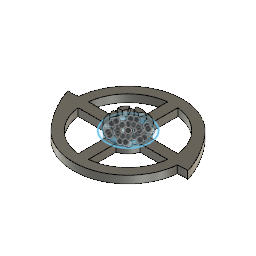
circular double tooth v9 (Autodesk Fusion 360 design; units mm, degrees)
Autodesk Fusion 360 part; units mm, degrees
note: some values were not read from the file. Set by a fixed rule: which sketch regions a step uses.
sketch "Sketch1" plane through (0, 0, 0) normal (0, 0, 1) x (1, 0, 0)
  circle A0 centre (0, 0) radius 2.95
  circle A1 centre (0, 0) radius 13.9
  circle A2 centre (0, 0) radius 50.5
  circle A3 centre (0, 0) radius 42.5
  line L0 (0, 0) -> (0, 50.5) construction
  line L1 (0, 0) -> (50, 0) construction
  line L2 (0, 0) -> (0, -50.5) construction
  line L3 (0, 0) -> (-50.5, 0) construction
  line L4 (0, -4) -> (-50.3413, -4)
  line L5 (0, 4) -> (-50.3413, 4)
  line L6 (0, 4) -> (50.3413, 4)
  line L7 (0, -4) -> (50.3413, -4)
  line L8 (-4, 0) -> (-4, 50)
  line L9 (4, 0) -> (4, 50)
  line L10 (4, 0) -> (4, -50)
  line L11 (-4, 0) -> (-4, -50)
  circle A4 centre (0, 0) radius 35
  spline S0 degree 5 poles (-50.3413, 4) (-50.1483, 3.3288) (-49.755, 2.0187) (-49.1428, 0.1498) (-48.2761, -2.1757) (-47.0702, -4.9467) (-45.6928, -7.7451) (-44.094, -10.7131) (-42.2399, -13.9102) (-40.1125, -17.3141) (-37.6988, -20.8633) (-35.5301, -23.7571) (-33.7651, -25.9282) (-32.5263, -27.3718) (-31.8913, -28.0927) knots 0 0 0 0 0 0 0.1 0.2 0.3 0.4 0.5 0.6 0.7 0.8 0.9 1 1 1 1 1 1
  line L12 (-51.0873, 6.594) -> (-49.5954, 1.406)
  line L13 (-33.7745, -25.9547) -> (-30.008, -30.2306)
  spline S1 degree 5 poles (-50.3413, 4) (-50.2904, 3.9577) (-50.1779, 3.8772) (-49.9773, 3.7688) (-49.645, 3.6492) (-49.1156, 3.5438) (-48.4657, 3.4848) (-47.6934, 3.4729) (-46.8065, 3.5051) (-45.8162, 3.5771) (-44.7343, 3.6845) (-43.8031, 3.7959) (-43.0704, 3.8929) (-42.5669, 3.9633) (-42.3113, 4) knots 0 0 0 0 0 0 0.1 0.2 0.3 0.4 0.5 0.6 0.7 0.8 0.9 1 1 1 1 1 1
  line L14 (-50.752, 4.3411) -> (-49.9307, 3.6589)
  line L15 (-43.3417, 3.852) -> (-41.281, 4.148)
  spline S2 degree 5 poles (50.3413, -4) (50.1483, -3.3288) (49.755, -2.0187) (49.1428, -0.1498) (48.2761, 2.1757) (47.0702, 4.9467) (45.6928, 7.7451) (44.094, 10.7131) (42.2399, 13.9102) (40.1125, 17.3141) (37.6988, 20.8633) (35.5301, 23.7571) (33.7651, 25.9282) (32.5263, 27.3718) (31.8913, 28.0927) knots 0 0 0 0 0 0 0.1 0.2 0.3 0.4 0.5 0.6 0.7 0.8 0.9 1 1 1 1 1 1
  line L16 (51.0873, -6.594) -> (49.5954, -1.406)
  line L17 (33.7745, 25.9547) -> (30.008, 30.2306)
  spline S3 degree 5 poles (50.3413, -4) (50.2904, -3.9577) (50.1779, -3.8772) (49.9773, -3.7688) (49.645, -3.6492) (49.1156, -3.5438) (48.4657, -3.4848) (47.6934, -3.4729) (46.8065, -3.5051) (45.8162, -3.5771) (44.7343, -3.6845) (43.8031, -3.7959) (43.0704, -3.8929) (42.5669, -3.9633) (42.3113, -4) knots 0 0 0 0 0 0 0.1 0.2 0.3 0.4 0.5 0.6 0.7 0.8 0.9 1 1 1 1 1 1
  line L18 (50.752, -4.3411) -> (49.9307, -3.6589)
  line L19 (43.3417, -3.852) -> (41.281, -4.148)
  point P0 (-45, -9)
  point P1 (-48.5, 3.5)
  point P2 (45, 9)
  point P3 (48.5, -3.5)
  dimension "d1" = 5.9
  dimension "d2" = 27.8
  dimension "d3" = 101
  dimension "d4" = 85
  dimension "d5" = 4
  dimension "d6" = 4
  dimension "d7" = 70
  constraint coincident A0.centre A1.centre
  constraint coincident A2 L0.end
  constraint vertical L0
  constraint perpendicular L0 L1
  constraint coincident A2 L2.end
  constraint vertical L2
  constraint coincident A2 L3.end
  constraint perpendicular L2 L3
  constraint coincident L2 L4.start
  constraint coincident A2 L4.end
  constraint perpendicular L2 L4
  constraint symmetric L3 L4.start L5.start
  constraint symmetric L3 L4.end L5.end
  constraint symmetric L0 L4.start L7.start
  constraint symmetric L0 L4.end L7.end
  constraint symmetric L0 L5.start L6.start
  constraint symmetric L0 L5.end L6.end
  constraint coincident L3 L8.start
  constraint perpendicular L3 L8
  constraint symmetric L0 L8.start L9.start
  constraint symmetric L0 L8.end L9.end
  constraint symmetric L1 L8.start L11.start
  constraint symmetric L1 L8.end L11.end
  constraint symmetric L1 L9.start L10.start
  constraint symmetric L1 L9.end L10.end
  constraint concentric A2 A4
  constraint midpoint L5.end L12
  constraint midpoint S0.end L13
  constraint coincident L5 S1.end
  constraint coincident A3 S1.end
  constraint midpoint L5.end L14
  constraint midpoint S1.end L15
  constraint coincident A3 S0.end
  constraint tangent A3 L13
  measures "d1" diameter of A0
  measures "d2" diameter of A1
  measures "d3" diameter of A2
  measures "d4" diameter of A3
  measures "d5" distance of L3 L4
  measures "d6" distance of L0 L8
  measures "d7" diameter of A4
extrude "Extrude1" add sketch "Sketch1" along normal mid plane 6 contours A1 L6 L7 L9 L10 | A1 L6 L7 A4 | A1 L6 L9 | A1 L7 L10 | A1 L5 L6 L8 L9 | A1 L8 L9 A4 | L4 L5 L6 L7 L8 L9 L10 L11 | A3 L6 L9 A4 | A3 L6 L7 A4 | A1 L10 L11 A4 | A1 L4 L7 L10 L11 | A3 L7 L10 A4 | A1 L5 L8 | A3 L8 L9 A4 | A3 L6 S2 S3 | A3 L6 S2 | A1 L4 L11 | A3 L10 L11 A4 | A1 L4 L5 L8 L11 | A1 L4 L5 A4 | A3 L5 L8 A4 | A3 L4 L11 A4 | A3 L4 L5 A4 | A3 L4 S0 S1 | A3 L4 S0
ref_plane "WorkPlane1" through (0, 0, 3) normal (0, 0, 1) x (1, 0, 0)
sketch "Sketch2" plane through (0, 0.1618, 3) normal (0, 0, 1) x (1, 0, 0)
  line L0 (-2.034, -6.023) -> (-4.3462, -10.0278)
  spline S0 degree 3 poles (-10.8574, -1.65) (-10.8584, -1.65) (-10.8595, -1.6501) (-10.8605, -1.6503) (-10.862, -1.6506) (-10.8635, -1.6511) (-10.8648, -1.6519) (-10.8666, -1.6528) (-10.8681, -1.654) (-10.8696, -1.6558) (-10.8707, -1.6572) (-10.8716, -1.6587) (-10.8722, -1.6607) (-10.8729, -1.6626) (-10.8731, -1.6646) (-10.873, -1.6667) knots -0.08749 -0.08749 -0.08749 -0.08749 -0.077534 -0.077534 -0.077534 -0.062667 -0.062667 -0.062667 -0.04351 -0.04351 -0.04351 -0.027229 -0.027229 -0.027229 -0.010666 -0.010666 -0.010666 -0.010666
  spline S1 degree 3 poles (-1.5005, -6.1547) (-1.5145, -6.1513) (-1.5288, -6.1496) (-1.5432, -6.1497) (-1.5589, -6.1497) (-1.5744, -6.1518) (-1.5895, -6.1559) (-1.6081, -6.161) (-1.6256, -6.169) (-1.6416, -6.1796) (-1.6557, -6.189) (-1.6683, -6.2003) (-1.6791, -6.2132) (-1.6837, -6.2186) (-1.6878, -6.2242) (-1.6917, -6.2301) knots -0.077702 -0.077702 -0.077702 -0.077702 -0.063693 -0.063693 -0.063693 -0.048454 -0.048454 -0.048454 -0.029774 -0.029774 -0.029774 -0.013339 -0.013339 -0.013339 -0.006509 -0.006509 -0.006509 -0.006509
  arc A0 (-4.2907, -4.1005) -> (-1.4057, -5.7661) centre (0, 0) ccw
  arc A1 (-11.2693, -1.7216) -> (-7.1256, -8.8987) centre (0, 0) ccw
  circle A2 centre (0, 0) radius 16.7005
  spline S2 degree 3 poles (-4.3462, -10.0278) (-4.349, -10.0327) (-4.3517, -10.0376) (-4.357, -10.0477) (-4.3595, -10.0528) (-4.3635, -10.0611) (-4.3649, -10.0643) (-4.3677, -10.0705) (-4.3689, -10.0734) (-4.3717, -10.0801) (-4.3732, -10.0838) (-4.3775, -10.0951) (-4.3801, -10.1027) (-4.3954, -10.1509) (-4.402, -10.1935) (-4.4018, -10.2542) (-4.4007, -10.2718) (-4.3915, -10.3419) (-4.3744, -10.3946) (-4.3231, -10.4833) (-4.2929, -10.5203) (-4.2227, -10.5801) (-4.185, -10.6033) (-4.1437, -10.6203) knots -0.079764 -0.079764 -0.079764 -0.079764 -0.077736 -0.077736 -0.075667 -0.075667 -0.074396 -0.074396 -0.073245 -0.073245 -0.071774 -0.071774 -0.068877 -0.068877 -0.053423 -0.053423 -0.047168 -0.047168 -0.028481 -0.028481 -0.013393 -0.013393 0 0 0 0
  spline S3 degree 3 poles (-10.8574, -1.25) (-10.8623, -1.25) (-10.8672, -1.2501) (-10.8783, -1.2505) (-10.8845, -1.2508) (-10.8945, -1.2516) (-10.8984, -1.252) (-10.9058, -1.2528) (-10.9094, -1.2532) (-10.9175, -1.2543) (-10.9221, -1.255) (-10.9363, -1.2574) (-10.9458, -1.2594) (-11.0105, -1.2751) (-11.063, -1.2998) (-11.1532, -1.3685) (-11.1916, -1.4115) (-11.2435, -1.5046) (-11.2601, -1.5511) (-11.2742, -1.6405) (-11.2748, -1.6811) (-11.2693, -1.7216) knots -0.086203 -0.086203 -0.086203 -0.086203 -0.084433 -0.084433 -0.082213 -0.082213 -0.08081 -0.08081 -0.079512 -0.079512 -0.077841 -0.077841 -0.0743 -0.0743 -0.053753 -0.053753 -0.034336 -0.034336 -0.018768 -0.018768 -0.006485 -0.006485 -0.006485 -0.006485
  spline S4 degree 3 poles (-5.6965, -1.6656) (-5.7165, -1.5973) (-5.7489, -1.5333) (-5.8314, -1.4253) (-5.8791, -1.3808) (-5.9816, -1.3132) (-6.0346, -1.2888) (-6.1368, -1.2591) (-6.1847, -1.2515) (-6.2331, -1.25) knots -0.072712 -0.072712 -0.072712 -0.072712 -0.051359 -0.051359 -0.031933 -0.031933 -0.014516 -0.014516 0 0 0 0
  circle A3 centre (0, 0) radius 6.1545
  spline S5 degree 3 poles (-6.8799, -8.583) (-6.8781, -8.5842) (-6.876, -8.585) (-6.874, -8.5853) (-6.8719, -8.5857) (-6.8702, -8.5857) (-6.8684, -8.5854) (-6.8665, -8.585) (-6.8649, -8.5844) (-6.8634, -8.5835) (-6.8623, -8.5829) (-6.8613, -8.5822) (-6.8604, -8.5813) (-6.8593, -8.5803) (-6.8584, -8.5791) (-6.8576, -8.5778) knots -0.146478 -0.146478 -0.146478 -0.146478 -0.128978 -0.128978 -0.128978 -0.112667 -0.112667 -0.112667 -0.096104 -0.096104 -0.096104 -0.084227 -0.084227 -0.084227 -0.069674 -0.069674 -0.069674 -0.069674
  line L1 (-6.2331, -1.25) -> (-10.8574, -1.25)
  spline S6 degree 3 poles (-3.9998, -10.2278) (-4.0003, -10.2287) (-4.0007, -10.2296) (-4.001, -10.2306) (-4.0015, -10.2321) (-4.0018, -10.2336) (-4.0018, -10.2352) (-4.0019, -10.2372) (-4.0016, -10.2391) (-4.0008, -10.2412) (-4.0002, -10.2429) (-3.9993, -10.2444) (-3.9979, -10.246) (-3.9966, -10.2475) (-3.995, -10.2487) (-3.9931, -10.2496) knots -0.08749 -0.08749 -0.08749 -0.08749 -0.077534 -0.077534 -0.077534 -0.062667 -0.062667 -0.062667 -0.04351 -0.04351 -0.04351 -0.027229 -0.027229 -0.027229 -0.010666 -0.010666 -0.010666 -0.010666
  arc A4 (-5.6965, 1.6656) -> (-5.6965, -1.6656) centre (0, 0) ccw
  circle A5 centre (0, 0) radius 2.7005
  line L2 (-6.8576, -8.5778) -> (-4.5496, -4.5801)
  line L3 (-6.2412, -1.65) -> (-10.8574, -1.65)
  line L4 (6.8576, 8.5778) -> (4.5496, 4.5801)
  spline S7 degree 3 poles (10.8574, 1.25) (10.8623, 1.25) (10.8672, 1.2501) (10.8783, 1.2505) (10.8845, 1.2508) (10.8945, 1.2516) (10.8984, 1.252) (10.9058, 1.2528) (10.9094, 1.2532) (10.9175, 1.2543) (10.9221, 1.255) (10.9363, 1.2574) (10.9458, 1.2594) (11.0105, 1.2751) (11.063, 1.2998) (11.1532, 1.3685) (11.1916, 1.4115) (11.2435, 1.5046) (11.2601, 1.5511) (11.2742, 1.6405) (11.2748, 1.6811) (11.2693, 1.7216) knots -0.086203 -0.086203 -0.086203 -0.086203 -0.084433 -0.084433 -0.082213 -0.082213 -0.08081 -0.08081 -0.079512 -0.079512 -0.077841 -0.077841 -0.0743 -0.0743 -0.053753 -0.053753 -0.034336 -0.034336 -0.018768 -0.018768 -0.006485 -0.006485 -0.006485 -0.006485
  line L5 (6.5112, 8.7778) -> (4.1991, 4.773)
  spline S8 degree 3 poles (7.1256, 8.8987) (7.1226, 8.9009) (7.1197, 8.9032) (7.0927, 8.9229) (7.0671, 8.9377) (6.9958, 8.9695) (6.9495, 8.9807) (6.8523, 8.9884) (6.8024, 8.9827) (6.7014, 8.9536) (6.6517, 8.9271) (6.5946, 8.8808) (6.5808, 8.8679) (6.5618, 8.8477) (6.5559, 8.8409) (6.5471, 8.8302) (6.544, 8.8263) (6.5385, 8.8191) (6.536, 8.8158) (6.5307, 8.8084) (6.5279, 8.8043) (6.5203, 8.7929) (6.5156, 8.7854) (6.5112, 8.7778) knots -0.080264 -0.080264 -0.080264 -0.080264 -0.079146 -0.079146 -0.070166 -0.070166 -0.055156 -0.055156 -0.03834 -0.03834 -0.018441 -0.018441 -0.011572 -0.011572 -0.008302 -0.008302 -0.006499 -0.006499 -0.004985 -0.004985 -0.003198 -0.003198 0 0 0 0
  arc A6 (4.1437, 10.6203) -> (-4.1437, 10.6203) centre (0, 0) ccw
  arc A7 (3.9931, 10.2496) -> (-3.9931, 10.2496) centre (0, 0) ccw
  spline S9 degree 3 poles (-4.1991, -4.773) (-4.1836, -4.7441) (-4.1705, -4.7138) (-4.1512, -4.6556) (-4.1442, -4.628) (-4.132, -4.5588) (-4.1293, -4.517) (-4.1337, -4.4126) (-4.1466, -4.3508) (-4.1966, -4.221) (-4.2379, -4.1557) (-4.2907, -4.1005) knots -0.072701 -0.072701 -0.072701 -0.072701 -0.062829 -0.062829 -0.054287 -0.054287 -0.041746 -0.041746 -0.02294 -0.02294 0 0 0 0
  spline S10 degree 3 poles (-4.1437, 10.6203) (-4.1757, 10.6071) (-4.2057, 10.5902) (-4.2631, 10.5478) (-4.2894, 10.5222) (-4.3436, 10.4539) (-4.3668, 10.4095) (-4.3963, 10.3184) (-4.4028, 10.2717) (-4.401, 10.1948) (-4.3968, 10.164) (-4.386, 10.1213) (-4.3822, 10.1087) (-4.376, 10.0912) (-4.3741, 10.0862) (-4.3709, 10.0781) (-4.3696, 10.0749) (-4.3669, 10.0688) (-4.3656, 10.0659) (-4.3626, 10.0592) (-4.3608, 10.0554) (-4.3551, 10.0438) (-4.3509, 10.0361) (-4.3464, 10.0282) (-4.3463, 10.028) (-4.3462, 10.0278) knots -0.099601 -0.099601 -0.099601 -0.099601 -0.089178 -0.089178 -0.077713 -0.077713 -0.061196 -0.061196 -0.044718 -0.044718 -0.033484 -0.033484 -0.028686 -0.028686 -0.026742 -0.026742 -0.025496 -0.025496 -0.024331 -0.024331 -0.022814 -0.022814 -0.019643 -0.019643 -0.019544 -0.019544 -0.019544 -0.019544
  spline S11 degree 3 poles (-6.2331, 1.25) (-6.1675, 1.2521) (-6.1027, 1.2653) (-6.0046, 1.3036) (-5.9692, 1.3217) (-5.8852, 1.3764) (-5.8399, 1.4173) (-5.7537, 1.5238) (-5.7179, 1.5923) (-5.6965, 1.6656) knots -0.072724 -0.072724 -0.072724 -0.072724 -0.05302 -0.05302 -0.041116 -0.041116 -0.022939 -0.022939 0 0 0 0
  spline S12 degree 3 poles (6.8799, 8.583) (6.8781, 8.5842) (6.876, 8.585) (6.874, 8.5853) (6.8719, 8.5857) (6.8702, 8.5857) (6.8684, 8.5854) (6.8665, 8.585) (6.8649, 8.5844) (6.8634, 8.5835) (6.8623, 8.5829) (6.8613, 8.5822) (6.8604, 8.5813) (6.8593, 8.5803) (6.8584, 8.5791) (6.8576, 8.5778) knots -0.146478 -0.146478 -0.146478 -0.146478 -0.128978 -0.128978 -0.128978 -0.112667 -0.112667 -0.112667 -0.096104 -0.096104 -0.096104 -0.084227 -0.084227 -0.084227 -0.069674 -0.069674 -0.069674 -0.069674
  arc A8 (-6.8799, 8.583) -> (-10.873, 1.6667) centre (0, 0) ccw
  line L6 (-3.9998, 10.2278) -> (-1.6917, 6.2301)
  line L7 (0, 1.65) -> (10.1158, 1.65)
  spline S13 degree 3 poles (1.4057, 5.7661) (1.4748, 5.7493) (1.5463, 5.7453) (1.681, 5.7627) (1.7434, 5.7818) (1.8533, 5.8367) (1.901, 5.8704) (1.9779, 5.9441) (2.0085, 5.9819) (2.034, 6.023) knots -0.072711 -0.072711 -0.072711 -0.072711 -0.051396 -0.051396 -0.031964 -0.031964 -0.014535 -0.014535 0 0 0 0
  line L8 (6.2412, 1.65) -> (10.8574, 1.65)
  circle A9 centre (0, 0) radius 6.335
  spline S14 degree 3 poles (-10.873, 1.6667) (-10.8731, 1.6645) (-10.8728, 1.6623) (-10.8721, 1.6604) (-10.8714, 1.6584) (-10.8705, 1.6569) (-10.8693, 1.6556) (-10.8681, 1.6541) (-10.8668, 1.653) (-10.8653, 1.6521) (-10.8642, 1.6515) (-10.863, 1.651) (-10.8619, 1.6507) (-10.8604, 1.6502) (-10.8589, 1.65) (-10.8574, 1.65) knots -0.146478 -0.146478 -0.146478 -0.146478 -0.128978 -0.128978 -0.128978 -0.112667 -0.112667 -0.112667 -0.096104 -0.096104 -0.096104 -0.084227 -0.084227 -0.084227 -0.069674 -0.069674 -0.069674 -0.069674
  arc A10 (-1.4057, 5.7661) -> (-4.2907, 4.1005) centre (0, 0) ccw
  line L9 (-4.1991, 4.773) -> (-6.5112, 8.7778)
  spline S15 degree 3 poles (-6.2412, 1.65) (-6.2226, 1.6511) (-6.2042, 1.6551) (-6.1868, 1.6619) (-6.1754, 1.6663) (-6.1645, 1.6719) (-6.1542, 1.6786) (-6.1386, 1.6888) (-6.1246, 1.7014) (-6.1129, 1.7159) (-6.0981, 1.7342) (-6.087, 1.7553) (-6.0804, 1.7779) knots -0.071247 -0.071247 -0.071247 -0.071247 -0.05302 -0.05302 -0.05302 -0.041116 -0.041116 -0.041116 -0.022939 -0.022939 -0.022939 0 0 0 0
  spline S16 degree 3 poles (-6.8576, 8.5778) (-6.8582, 8.5787) (-6.8588, 8.5795) (-6.8594, 8.5803) (-6.8605, 8.5815) (-6.8617, 8.5825) (-6.863, 8.5833) (-6.8647, 8.5843) (-6.8665, 8.5851) (-6.8687, 8.5854) (-6.8705, 8.5857) (-6.8723, 8.5857) (-6.8743, 8.5853) (-6.8763, 8.5849) (-6.8782, 8.5841) (-6.8799, 8.583) knots -0.08749 -0.08749 -0.08749 -0.08749 -0.077534 -0.077534 -0.077534 -0.062667 -0.062667 -0.062667 -0.04351 -0.04351 -0.04351 -0.027229 -0.027229 -0.027229 -0.010666 -0.010666 -0.010666 -0.010666
  arc A11 (4.2907, 4.1005) -> (1.4057, 5.7661) centre (0, 0) ccw
  spline S17 degree 3 poles (4.5496, 4.5801) (4.5412, 4.5634) (4.5354, 4.5455) (4.5326, 4.527) (4.5307, 4.5149) (4.5301, 4.5026) (4.5308, 4.4904) (4.5318, 4.4718) (4.5357, 4.4534) (4.5424, 4.436) (4.5509, 4.414) (4.5636, 4.3939) (4.5799, 4.3768) knots -0.071247 -0.071247 -0.071247 -0.071247 -0.05302 -0.05302 -0.05302 -0.041116 -0.041116 -0.041116 -0.022939 -0.022939 -0.022939 0 0 0 0
  spline S18 degree 3 poles (6.0804, 1.7779) (6.0844, 1.7641) (6.0901, 1.7508) (6.0974, 1.7384) (6.1052, 1.7248) (6.1149, 1.7124) (6.126, 1.7014) (6.1396, 1.6879) (6.1553, 1.6766) (6.1725, 1.6681) (6.1877, 1.6607) (6.2038, 1.6554) (6.2204, 1.6524) (6.2273, 1.6512) (6.2343, 1.6504) (6.2412, 1.65) knots -0.077702 -0.077702 -0.077702 -0.077702 -0.063693 -0.063693 -0.063693 -0.048454 -0.048454 -0.048454 -0.029774 -0.029774 -0.029774 -0.013339 -0.013339 -0.013339 -0.006509 -0.006509 -0.006509 -0.006509
  spline S19 degree 3 poles (-2.034, 6.023) (-1.9994, 5.9673) (-1.9556, 5.9178) (-1.8735, 5.852) (-1.84, 5.8304) (-1.7506, 5.7849) (-1.6926, 5.7661) (-1.5572, 5.7448) (-1.48, 5.748) (-1.4057, 5.7661) knots -0.072724 -0.072724 -0.072724 -0.072724 -0.053033 -0.053033 -0.041123 -0.041123 -0.02294 -0.02294 0 0 0 0
  spline S20 degree 3 poles (3.9998, 10.2278) (4.0003, 10.2287) (4.0007, 10.2296) (4.001, 10.2306) (4.0015, 10.2321) (4.0018, 10.2336) (4.0018, 10.2352) (4.0019, 10.2372) (4.0016, 10.2391) (4.0008, 10.2412) (4.0002, 10.2429) (3.9993, 10.2444) (3.9979, 10.246) (3.9966, 10.2475) (3.995, 10.2487) (3.9931, 10.2496) knots -0.08749 -0.08749 -0.08749 -0.08749 -0.077534 -0.077534 -0.077534 -0.062667 -0.062667 -0.062667 -0.04351 -0.04351 -0.04351 -0.027229 -0.027229 -0.027229 -0.010666 -0.010666 -0.010666 -0.010666
  spline S21 degree 3 poles (4.3462, 10.0278) (4.349, 10.0327) (4.3517, 10.0376) (4.357, 10.0477) (4.3595, 10.0528) (4.3635, 10.0611) (4.3649, 10.0643) (4.3677, 10.0705) (4.3689, 10.0734) (4.3717, 10.0801) (4.3732, 10.0838) (4.3775, 10.0951) (4.3801, 10.1027) (4.3954, 10.1509) (4.402, 10.1935) (4.4018, 10.2542) (4.4007, 10.2718) (4.3915, 10.3419) (4.3744, 10.3946) (4.3231, 10.4833) (4.2929, 10.5203) (4.2227, 10.5801) (4.185, 10.6033) (4.1437, 10.6203) knots -0.079764 -0.079764 -0.079764 -0.079764 -0.077736 -0.077736 -0.075667 -0.075667 -0.074396 -0.074396 -0.073245 -0.073245 -0.071774 -0.071774 -0.068877 -0.068877 -0.053423 -0.053423 -0.047168 -0.047168 -0.028481 -0.028481 -0.013393 -0.013393 0 0 0 0
  spline S22 degree 3 poles (1.5005, 6.1547) (1.5145, 6.1513) (1.5288, 6.1496) (1.5432, 6.1497) (1.5589, 6.1497) (1.5744, 6.1518) (1.5895, 6.1559) (1.6081, 6.161) (1.6256, 6.169) (1.6416, 6.1796) (1.6557, 6.189) (1.6683, 6.2003) (1.6791, 6.2132) (1.6837, 6.2186) (1.6878, 6.2242) (1.6917, 6.2301) knots -0.077702 -0.077702 -0.077702 -0.077702 -0.063693 -0.063693 -0.063693 -0.048454 -0.048454 -0.048454 -0.029774 -0.029774 -0.029774 -0.013339 -0.013339 -0.013339 -0.006509 -0.006509 -0.006509 -0.006509
  line L10 (2.034, 6.023) -> (4.3462, 10.0278)
  spline S23 degree 3 poles (4.1991, 4.773) (4.1836, 4.7441) (4.1705, 4.7138) (4.1512, 4.6556) (4.1442, 4.628) (4.132, 4.5588) (4.1293, 4.517) (4.1337, 4.4126) (4.1466, 4.3508) (4.1966, 4.221) (4.2379, 4.1557) (4.2907, 4.1005) knots -0.072701 -0.072701 -0.072701 -0.072701 -0.062829 -0.062829 -0.054287 -0.054287 -0.041746 -0.041746 -0.02294 -0.02294 0 0 0 0
  spline S24 degree 3 poles (-11.2693, 1.7216) (-11.272, 1.7015) (-11.2732, 1.6813) (-11.2725, 1.6136) (-11.2639, 1.5679) (-11.2314, 1.4771) (-11.2059, 1.4341) (-11.1436, 1.3604) (-11.1068, 1.3299) (-11.0381, 1.2899) (-11.0078, 1.2768) (-10.9639, 1.2637) (-10.9512, 1.2605) (-10.9321, 1.2567) (-10.9258, 1.2556) (-10.9155, 1.2541) (-10.9116, 1.2535) (-10.9042, 1.2526) (-10.9006, 1.2522) (-10.8925, 1.2515) (-10.8879, 1.2511) (-10.8747, 1.2503) (-10.8661, 1.25) (-10.8574, 1.25) knots -0.149421 -0.149421 -0.149421 -0.149421 -0.143292 -0.143292 -0.128978 -0.128978 -0.112667 -0.112667 -0.096104 -0.096104 -0.084227 -0.084227 -0.079495 -0.079495 -0.07717 -0.07717 -0.075742 -0.075742 -0.074448 -0.074448 -0.072794 -0.072794 -0.069674 -0.069674 -0.069674 -0.069674
  arc A12 (10.873, 1.6667) -> (6.8799, 8.583) centre (0, 0) ccw
  spline S25 degree 3 poles (-6.5112, 8.7778) (-6.5152, 8.7846) (-6.5193, 8.7914) (-6.526, 8.8015) (-6.5283, 8.8049) (-6.5332, 8.8119) (-6.5356, 8.8153) (-6.5409, 8.8223) (-6.5436, 8.8258) (-6.5506, 8.8345) (-6.5549, 8.8397) (-6.571, 8.858) (-6.5835, 8.8704) (-6.6143, 8.8975) (-6.6332, 8.9116) (-6.6989, 8.952) (-6.7506, 8.9717) (-6.8537, 8.988) (-6.9038, 8.9875) (-6.9977, 8.9684) (-7.0406, 8.9524) (-7.0964, 8.9198) (-7.1114, 8.9097) (-7.1256, 8.8987) knots -0.08749 -0.08749 -0.08749 -0.08749 -0.084639 -0.084639 -0.083129 -0.083129 -0.081593 -0.081593 -0.079982 -0.079982 -0.077534 -0.077534 -0.071156 -0.071156 -0.062667 -0.062667 -0.04351 -0.04351 -0.027229 -0.027229 -0.013166 -0.013166 -0.007722 -0.007722 -0.007722 -0.007722
  line L11 (1.6917, 6.2301) -> (3.9998, 10.2278)
  line L12 (6.2331, 1.25) -> (10.8574, 1.25)
  line L13 (-10.8574, 1.25) -> (-6.2331, 1.25)
  line L14 (-4.3462, 10.0278) -> (-2.034, 6.023)
  spline S26 degree 3 poles (5.6965, 1.6656) (5.7165, 1.5973) (5.7489, 1.5333) (5.8314, 1.4253) (5.8791, 1.3808) (5.9816, 1.3132) (6.0346, 1.2888) (6.1368, 1.2591) (6.1847, 1.2515) (6.2331, 1.25) knots -0.072712 -0.072712 -0.072712 -0.072712 -0.051359 -0.051359 -0.031933 -0.031933 -0.014516 -0.014516 0 0 0 0
  arc A13 (11.2693, 1.7216) -> (7.1256, 8.8987) centre (0, 0) ccw
  spline S27 degree 3 poles (10.8574, 1.65) (10.8584, 1.65) (10.8595, 1.6501) (10.8605, 1.6503) (10.862, 1.6506) (10.8635, 1.6511) (10.8648, 1.6519) (10.8666, 1.6528) (10.8681, 1.654) (10.8696, 1.6558) (10.8707, 1.6572) (10.8716, 1.6587) (10.8722, 1.6607) (10.8729, 1.6626) (10.8731, 1.6646) (10.873, 1.6667) knots -0.08749 -0.08749 -0.08749 -0.08749 -0.077534 -0.077534 -0.077534 -0.062667 -0.062667 -0.062667 -0.04351 -0.04351 -0.04351 -0.027229 -0.027229 -0.027229 -0.010666 -0.010666 -0.010666 -0.010666
  spline S28 degree 3 poles (-4.2907, 4.1005) (-4.2585, 4.1342) (-4.2304, 4.1718) (-4.1819, 4.2563) (-4.1626, 4.3035) (-4.1338, 4.4129) (-4.1277, 4.4752) (-4.1353, 4.592) (-4.1466, 4.6459) (-4.1747, 4.7234) (-4.186, 4.7486) (-4.1991, 4.773) knots -0.077702 -0.077702 -0.077702 -0.077702 -0.063693 -0.063693 -0.048454 -0.048454 -0.029774 -0.029774 -0.013339 -0.013339 -0.00503 -0.00503 -0.00503 -0.00503
  line L15 (-4.5496, 4.5801) -> (-6.8576, 8.5778)
  spline S29 degree 3 poles (-3.9931, 10.2496) (-3.9951, 10.2487) (-3.9968, 10.2473) (-3.9981, 10.2457) (-3.9995, 10.2441) (-4.0003, 10.2426) (-4.0009, 10.2409) (-4.0016, 10.2391) (-4.0018, 10.2374) (-4.0018, 10.2357) (-4.0019, 10.2344) (-4.0017, 10.2332) (-4.0014, 10.232) (-4.0011, 10.2305) (-4.0005, 10.2291) (-3.9998, 10.2278) knots -0.146478 -0.146478 -0.146478 -0.146478 -0.128978 -0.128978 -0.128978 -0.112667 -0.112667 -0.112667 -0.096104 -0.096104 -0.096104 -0.084227 -0.084227 -0.084227 -0.069674 -0.069674 -0.069674 -0.069674
  spline S30 degree 3 poles (-4.5799, 4.3768) (-4.57, 4.3872) (-4.5613, 4.3988) (-4.5542, 4.4113) (-4.5464, 4.4249) (-4.5404, 4.4394) (-4.5364, 4.4546) (-4.5315, 4.4731) (-4.5297, 4.4923) (-4.5309, 4.5115) (-4.532, 4.5283) (-4.5355, 4.5449) (-4.5412, 4.5608) (-4.5436, 4.5674) (-4.5464, 4.5738) (-4.5496, 4.5801) knots -0.077702 -0.077702 -0.077702 -0.077702 -0.063693 -0.063693 -0.063693 -0.048454 -0.048454 -0.048454 -0.029774 -0.029774 -0.029774 -0.013339 -0.013339 -0.013339 -0.006509 -0.006509 -0.006509 -0.006509
  spline S31 degree 3 poles (-1.6917, 6.2301) (-1.6814, 6.2144) (-1.6688, 6.2005) (-1.6542, 6.1888) (-1.6446, 6.1812) (-1.6343, 6.1745) (-1.6234, 6.169) (-1.6068, 6.1605) (-1.5889, 6.1547) (-1.5704, 6.1518) (-1.5472, 6.1482) (-1.5234, 6.1492) (-1.5005, 6.1547) knots -0.071247 -0.071247 -0.071247 -0.071247 -0.05302 -0.05302 -0.05302 -0.041116 -0.041116 -0.041116 -0.022939 -0.022939 -0.022939 0 0 0 0
  line L16 (-10.8574, 1.65) -> (-6.2412, 1.65)
  circle A14 centre (0, 0) radius 2.7
  arc A15 (8.9156, 8.7614) -> (-10.9659, 6) centre (0, 0) ccw
  arc A16 (-7.1256, 8.8987) -> (-11.2693, 1.7216) centre (0, 0) ccw
  arc A17 (-10.9659, -6) -> (8.9156, -8.7614) centre (0, 0) ccw
  spline S32 degree 3 poles (6.8576, -8.5778) (6.8582, -8.5787) (6.8588, -8.5795) (6.8594, -8.5803) (6.8605, -8.5815) (6.8617, -8.5825) (6.863, -8.5833) (6.8647, -8.5843) (6.8665, -8.5851) (6.8687, -8.5854) (6.8705, -8.5857) (6.8723, -8.5857) (6.8743, -8.5853) (6.8763, -8.5849) (6.8782, -8.5841) (6.8799, -8.583) knots -0.08749 -0.08749 -0.08749 -0.08749 -0.077534 -0.077534 -0.077534 -0.062667 -0.062667 -0.062667 -0.04351 -0.04351 -0.04351 -0.027229 -0.027229 -0.027229 -0.010666 -0.010666 -0.010666 -0.010666
  arc A18 (-3.9931, -10.2496) -> (3.9931, -10.2496) centre (0, 0) ccw
  arc A19 (5.6965, -1.6656) -> (5.6965, 1.6656) centre (0, 0) ccw
  arc A20 (-4.1437, -10.6203) -> (4.1437, -10.6203) centre (0, 0) ccw
  circle A21 centre (0, 0) radius 10.2495
  spline S33 degree 3 poles (2.034, -6.023) (1.9994, -5.9673) (1.9556, -5.9178) (1.8735, -5.852) (1.84, -5.8304) (1.7506, -5.7849) (1.6926, -5.7661) (1.5572, -5.7448) (1.48, -5.748) (1.4057, -5.7661) knots -0.072724 -0.072724 -0.072724 -0.072724 -0.053033 -0.053033 -0.041123 -0.041123 -0.02294 -0.02294 0 0 0 0
  arc A22 (-10.873, -1.6667) -> (-6.8799, -8.583) centre (0, 0) ccw
  line L17 (-1.6917, -6.2301) -> (-3.9998, -10.2278)
  spline S34 degree 3 poles (6.5112, -8.7778) (6.5152, -8.7846) (6.5193, -8.7914) (6.526, -8.8015) (6.5283, -8.8049) (6.5332, -8.8119) (6.5356, -8.8153) (6.5409, -8.8223) (6.5436, -8.8258) (6.5506, -8.8345) (6.5549, -8.8397) (6.571, -8.858) (6.5835, -8.8704) (6.6143, -8.8975) (6.6332, -8.9116) (6.6989, -8.952) (6.7506, -8.9717) (6.8537, -8.988) (6.9038, -8.9875) (6.9977, -8.9684) (7.0406, -8.9524) (7.0964, -8.9198) (7.1114, -8.9097) (7.1256, -8.8987) knots -0.08749 -0.08749 -0.08749 -0.08749 -0.084639 -0.084639 -0.083129 -0.083129 -0.081593 -0.081593 -0.079982 -0.079982 -0.077534 -0.077534 -0.071156 -0.071156 -0.062667 -0.062667 -0.04351 -0.04351 -0.027229 -0.027229 -0.013166 -0.013166 -0.007722 -0.007722 -0.007722 -0.007722
  spline S35 degree 3 poles (-7.1256, -8.8987) (-7.1226, -8.9009) (-7.1197, -8.9032) (-7.0927, -8.9229) (-7.0671, -8.9377) (-6.9958, -8.9695) (-6.9495, -8.9807) (-6.8523, -8.9884) (-6.8024, -8.9827) (-6.7014, -8.9536) (-6.6517, -8.9271) (-6.5946, -8.8808) (-6.5808, -8.8679) (-6.5618, -8.8477) (-6.5559, -8.8409) (-6.5471, -8.8302) (-6.544, -8.8263) (-6.5385, -8.8191) (-6.536, -8.8158) (-6.5307, -8.8084) (-6.5279, -8.8043) (-6.5203, -8.7929) (-6.5156, -8.7854) (-6.5112, -8.7778) knots -0.080264 -0.080264 -0.080264 -0.080264 -0.079146 -0.079146 -0.070166 -0.070166 -0.055156 -0.055156 -0.03834 -0.03834 -0.018441 -0.018441 -0.011572 -0.011572 -0.008302 -0.008302 -0.006499 -0.006499 -0.004985 -0.004985 -0.003198 -0.003198 0 0 0 0
  arc A23 (7.1256, -8.8987) -> (11.2693, -1.7216) centre (0, 0) ccw
  spline S36 degree 3 poles (4.2907, -4.1005) (4.2585, -4.1342) (4.2304, -4.1718) (4.1819, -4.2563) (4.1626, -4.3035) (4.1338, -4.4129) (4.1277, -4.4752) (4.1353, -4.592) (4.1466, -4.6459) (4.1747, -4.7234) (4.186, -4.7486) (4.1991, -4.773) knots -0.077702 -0.077702 -0.077702 -0.077702 -0.063693 -0.063693 -0.048454 -0.048454 -0.029774 -0.029774 -0.013339 -0.013339 -0.00503 -0.00503 -0.00503 -0.00503
  spline S37 degree 3 poles (6.2412, -1.65) (6.2226, -1.6511) (6.2042, -1.6551) (6.1868, -1.6619) (6.1754, -1.6663) (6.1645, -1.6719) (6.1542, -1.6786) (6.1386, -1.6888) (6.1246, -1.7014) (6.1129, -1.7159) (6.0981, -1.7342) (6.087, -1.7553) (6.0804, -1.7779) knots -0.071247 -0.071247 -0.071247 -0.071247 -0.05302 -0.05302 -0.05302 -0.041116 -0.041116 -0.041116 -0.022939 -0.022939 -0.022939 0 0 0 0
  spline S38 degree 3 poles (10.873, -1.6667) (10.8731, -1.6645) (10.8728, -1.6623) (10.8721, -1.6604) (10.8714, -1.6584) (10.8705, -1.6569) (10.8693, -1.6556) (10.8681, -1.6541) (10.8668, -1.653) (10.8653, -1.6521) (10.8642, -1.6515) (10.863, -1.651) (10.8619, -1.6507) (10.8604, -1.6502) (10.8589, -1.65) (10.8574, -1.65) knots -0.146478 -0.146478 -0.146478 -0.146478 -0.128978 -0.128978 -0.128978 -0.112667 -0.112667 -0.112667 -0.096104 -0.096104 -0.096104 -0.084227 -0.084227 -0.084227 -0.069674 -0.069674 -0.069674 -0.069674
  spline S39 degree 3 poles (11.2693, -1.7216) (11.272, -1.7015) (11.2732, -1.6813) (11.2725, -1.6136) (11.2639, -1.5679) (11.2314, -1.4771) (11.2059, -1.4341) (11.1436, -1.3604) (11.1068, -1.3299) (11.0381, -1.2899) (11.0078, -1.2768) (10.9639, -1.2637) (10.9512, -1.2605) (10.9321, -1.2567) (10.9258, -1.2556) (10.9155, -1.2541) (10.9116, -1.2535) (10.9042, -1.2526) (10.9006, -1.2522) (10.8925, -1.2515) (10.8879, -1.2511) (10.8747, -1.2503) (10.8661, -1.25) (10.8574, -1.25) knots -0.149421 -0.149421 -0.149421 -0.149421 -0.143292 -0.143292 -0.128978 -0.128978 -0.112667 -0.112667 -0.096104 -0.096104 -0.084227 -0.084227 -0.079495 -0.079495 -0.07717 -0.07717 -0.075742 -0.075742 -0.074448 -0.074448 -0.072794 -0.072794 -0.069674 -0.069674 -0.069674 -0.069674
  arc A24 (6.8799, -8.583) -> (10.873, -1.6667) centre (0, 0) ccw
  spline S40 degree 3 poles (-6.0804, -1.7779) (-6.0844, -1.7641) (-6.0901, -1.7508) (-6.0974, -1.7384) (-6.1052, -1.7248) (-6.1149, -1.7124) (-6.126, -1.7014) (-6.1396, -1.6879) (-6.1553, -1.6766) (-6.1725, -1.6681) (-6.1877, -1.6607) (-6.2038, -1.6554) (-6.2204, -1.6524) (-6.2273, -1.6512) (-6.2343, -1.6504) (-6.2412, -1.65) knots -0.077702 -0.077702 -0.077702 -0.077702 -0.063693 -0.063693 -0.063693 -0.048454 -0.048454 -0.048454 -0.029774 -0.029774 -0.029774 -0.013339 -0.013339 -0.013339 -0.006509 -0.006509 -0.006509 -0.006509
  spline S41 degree 3 poles (4.5799, -4.3768) (4.57, -4.3872) (4.5613, -4.3988) (4.5542, -4.4113) (4.5464, -4.4249) (4.5404, -4.4394) (4.5364, -4.4546) (4.5315, -4.4731) (4.5297, -4.4923) (4.5309, -4.5115) (4.532, -4.5283) (4.5355, -4.5449) (4.5412, -4.5608) (4.5436, -4.5674) (4.5464, -4.5738) (4.5496, -4.5801) knots -0.077702 -0.077702 -0.077702 -0.077702 -0.063693 -0.063693 -0.063693 -0.048454 -0.048454 -0.048454 -0.029774 -0.029774 -0.029774 -0.013339 -0.013339 -0.013339 -0.006509 -0.006509 -0.006509 -0.006509
  spline S42 degree 3 poles (4.1437, -10.6203) (4.1757, -10.6071) (4.2057, -10.5902) (4.2631, -10.5478) (4.2894, -10.5222) (4.3436, -10.4539) (4.3668, -10.4095) (4.3963, -10.3184) (4.4028, -10.2717) (4.401, -10.1948) (4.3968, -10.164) (4.386, -10.1213) (4.3822, -10.1087) (4.376, -10.0912) (4.3741, -10.0862) (4.3709, -10.0781) (4.3696, -10.0749) (4.3669, -10.0688) (4.3656, -10.0659) (4.3626, -10.0592) (4.3608, -10.0554) (4.3551, -10.0438) (4.3509, -10.0361) (4.3464, -10.0282) (4.3463, -10.028) (4.3462, -10.0278) knots -0.099601 -0.099601 -0.099601 -0.099601 -0.089178 -0.089178 -0.077713 -0.077713 -0.061196 -0.061196 -0.044718 -0.044718 -0.033484 -0.033484 -0.028686 -0.028686 -0.026742 -0.026742 -0.025496 -0.025496 -0.024331 -0.024331 -0.022814 -0.022814 -0.019643 -0.019643 -0.019544 -0.019544 -0.019544 -0.019544
  line L18 (4.5496, -4.5801) -> (6.8576, -8.5778)
  line L19 (3.9998, -10.2278) -> (1.6917, -6.2301)
  spline S43 degree 3 poles (-1.4057, -5.7661) (-1.4298, -5.7603) (-1.4542, -5.7559) (-1.5247, -5.7481) (-1.571, -5.7485) (-1.681, -5.7627) (-1.7434, -5.7818) (-1.8533, -5.8367) (-1.901, -5.8704) (-1.9779, -5.9441) (-2.0085, -5.9819) (-2.034, -6.023) knots -0.072677 -0.072677 -0.072677 -0.072677 -0.065242 -0.065242 -0.051396 -0.051396 -0.031964 -0.031964 -0.014535 -0.014535 0 0 0 0
  circle A25 centre (0, 0) radius 13.9
  line L20 (4.3462, -10.0278) -> (2.034, -6.023)
  arc A26 (1.4057, -5.7661) -> (4.2907, -4.1005) centre (0, 0) ccw
  circle A27 centre (0, 0) radius 5.935
  spline S44 degree 3 poles (-4.5496, -4.5801) (-4.5412, -4.5634) (-4.5354, -4.5455) (-4.5326, -4.527) (-4.5307, -4.5149) (-4.5301, -4.5026) (-4.5308, -4.4904) (-4.5318, -4.4718) (-4.5357, -4.4534) (-4.5424, -4.436) (-4.5509, -4.414) (-4.5636, -4.3939) (-4.5799, -4.3768) knots -0.071247 -0.071247 -0.071247 -0.071247 -0.05302 -0.05302 -0.05302 -0.041116 -0.041116 -0.041116 -0.022939 -0.022939 -0.022939 0 0 0 0
  spline S45 degree 3 poles (6.2331, -1.25) (6.1675, -1.2521) (6.1027, -1.2653) (6.0046, -1.3036) (5.9692, -1.3217) (5.8852, -1.3764) (5.8399, -1.4173) (5.7537, -1.5238) (5.7179, -1.5923) (5.6965, -1.6656) knots -0.072724 -0.072724 -0.072724 -0.072724 -0.05302 -0.05302 -0.041116 -0.041116 -0.022939 -0.022939 0 0 0 0
  spline S46 degree 3 poles (1.6917, -6.2301) (1.6814, -6.2144) (1.6688, -6.2005) (1.6542, -6.1888) (1.6446, -6.1812) (1.6343, -6.1745) (1.6234, -6.169) (1.6068, -6.1605) (1.5889, -6.1547) (1.5704, -6.1518) (1.5472, -6.1482) (1.5234, -6.1492) (1.5005, -6.1547) knots -0.071247 -0.071247 -0.071247 -0.071247 -0.05302 -0.05302 -0.05302 -0.041116 -0.041116 -0.041116 -0.022939 -0.022939 -0.022939 0 0 0 0
  line L21 (10.8574, -1.65) -> (6.2412, -1.65)
  line L22 (4.1991, -4.773) -> (6.5112, -8.7778)
  spline S47 degree 3 poles (3.9931, -10.2496) (3.9951, -10.2487) (3.9968, -10.2473) (3.9981, -10.2457) (3.9995, -10.2441) (4.0003, -10.2426) (4.0009, -10.2409) (4.0016, -10.2391) (4.0018, -10.2374) (4.0018, -10.2357) (4.0019, -10.2344) (4.0017, -10.2332) (4.0014, -10.232) (4.0011, -10.2305) (4.0005, -10.2291) (3.9998, -10.2278) knots -0.146478 -0.146478 -0.146478 -0.146478 -0.128978 -0.128978 -0.128978 -0.112667 -0.112667 -0.112667 -0.096104 -0.096104 -0.096104 -0.084227 -0.084227 -0.084227 -0.069674 -0.069674 -0.069674 -0.069674
  line L23 (-6.5112, -8.7778) -> (-4.1991, -4.773)
  line L24 (10.8574, -1.25) -> (6.2331, -1.25)
  dimension "d13" = -0.4
  dimension "d14" = 360
  constraint coincident A0.centre A1.centre
  constraint concentric A19 A27
  constraint concentric A9 A27
  constraint coincident S30.start A9
extrude "Extrude2" add sketch "Sketch2" along normal blind 9.5 contours S1 A9 A21 L17 L19 S46 | L2 L3 A9 A21 S40 S44 | A9 A21 S37 S41 L18 L21 | A9 S15 L15 S30 L16 A21 | L6 A9 S22 L11 S31 A21 | L4 L7 L8 A9 S17 S18 A21
extrude "Extrude3" add sketch "Sketch2" along normal blind 5 contours L0 S1 A9 A21 L17 | L0 A9 A21 L23 | A3 A9 S33 S43 | A3 S9 A9 S43 | S47 | S6 | L0 S2 A18 A20 A21 L17 S42 L19 L20 | S4 A3 S9 A9 | L2 A9 A21 S44 L23 | A3 S33 S43 A27 | A0 A3 S9 S43 A27 | S5 | S0 | A1 S3 L1 L2 L3 A21 A22 S35 L23 | A18 A21 L17 L19 | S4 A3 S9 A27 | A9 A21 L19 L20 S46 | A3 S33 S36 A26 A27 | A3 A9 S33 S36 | A0 A4 A10 A11 A19 A26 A27 | L2 L3 A21 A22 | S4 A3 A4 S11 A27 | S4 A3 S11 A9 | L1 L3 A9 A21 S40 | A9 A21 L20 L22 | A3 S36 A27 S45 | A3 A9 S36 S45 | L1 A9 L13 A21 | A3 S11 A9 S28 | A3 S11 S28 A27 | A9 A21 S41 L18 L22 | A3 S26 A19 A27 S45 | A3 A9 S26 S45 | S38 | S32 | A21 S34 A23 S39 A24 L18 L21 L22 L24 | A9 S15 L13 L16 A21 | A3 A9 S19 S28 | A3 A10 S19 S28 A27 | A9 A21 S37 L21 L24 | A9 L12 A21 L24 | S14 | S16 | A8 L9 S24 S25 L13 L15 L16 A16 A21 | A21 A24 L18 L21 | A3 S13 A9 S19 | A3 S13 S19 A27 | A9 L9 L14 A21 | A9 L9 L15 S30 A21 | A3 L7 S26 | A3 L7 A9 S26 | A8 L15 L16 A21 | A3 S13 A9 S23 | A3 S13 A11 S23 A27 | L6 A9 L14 S31 A21 | A3 L7 S23 A27 | A3 L7 A9 S23 | L7 L8 A9 L12 A21 | L5 A9 L10 A21 | A9 S22 L10 L11 A21 | S29 | S20 | A6 A7 S10 L6 S21 L10 L11 L14 A21 | L7 A9 S18 | S12 | S27 | L4 S7 L5 S8 L8 A12 L12 A13 A21 | L4 L5 A9 S17 A21 | A7 L6 L11 A21 | L4 L8 A12 A21 | A5 A14 | A25
extrude "Extrude4" cut sketch "Sketch2" along normal blind 9.5 contours A5 A14
